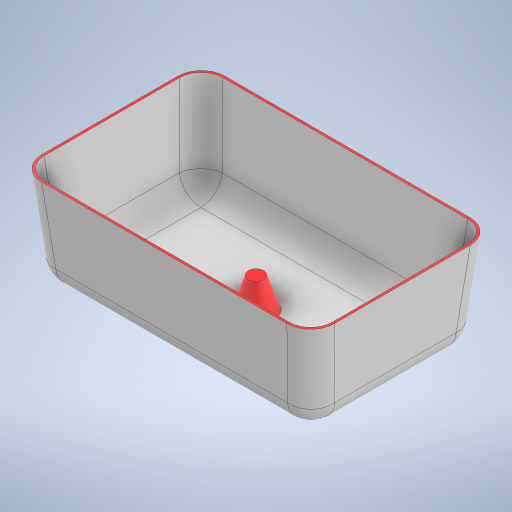
# Autodesk Inventor part: ContenedorBase
Saved by Autodesk Inventor 2024 (Build 280153000, 153)
## iProperties
Created: 2024-05-29
Part Number: ContenedorBase
Material: Genérico
Document SubType Name: Modeling
Designer: alexa
Density: 1 g/cm^3
Appearance: Valor por defecto
Author: alexa
Autodesk Inventor part; units mm, degrees
ref_plane "YZ Plane" through (0, 0, 0) normal (1, 0, 0) x (0, 1, 0)
sketch "Sketch1" plane through (0, 0, 0) normal (0, 1, 0) x (-1, 0, 0)
  line L0 (-57.75, 34.55) -> (57.75, 34.55)
  line L1 (57.75, 34.55) -> (57.75, -34.55)
  line L2 (57.75, -34.55) -> (-57.75, -34.55)
  line L3 (-57.75, -34.55) -> (-57.75, 34.55)
  line L4 (-57.75, 34.55) -> (57.75, -34.55) construction
  line L5 (57.75, 34.55) -> (-57.75, -34.55) construction
  point P0 (0, 0)
  dimension "d0" = 115.5
  dimension "d1" = 69.1
  constraints: 12 end point, 2 midpoint, 2 parallel, 1 horizontal, 1 perpendicular
  measures "d0" distance of L1.end L2.end
  measures "d1" distance of L0.end L1.end
ref_plane "Work Plane1" through (0, 40.8, 0) normal (0, 1, 0) x (-1, 0, 0)
sketch "Sketch2" plane through (0, 40.8, 0) normal (0, 1, 0) x (-1, 0, 0)
  line L0 (-61.45, 38.5) -> (61.45, 38.5)
  line L1 (61.45, 38.5) -> (61.45, -38.5)
  line L2 (61.45, -38.5) -> (-61.45, -38.5)
  line L3 (-61.45, -38.5) -> (-61.45, 38.5)
  line L4 (-61.45, 38.5) -> (61.45, -38.5) construction
  line L5 (61.45, 38.5) -> (-61.45, -38.5) construction
  point P0 (0, 0)
  dimension "d3" = 122.9
  dimension "d4" = 77
  constraints: 12 end point, 2 midpoint, 2 parallel, 1 horizontal, 1 perpendicular
  measures "d3" distance of L1.end L2.end
  measures "d4" distance of L0.end L1.end
loft "Loft1" add profiles "Sketch1", "Sketch2"
fillet "Fillet1" radius 10 8 edges at (59.6, 20.4, 36.525) (59.6, 20.4, -36.525) (-59.6, 20.4, 36.525) (-59.6, 20.4, -36.525) (0, 0, -34.55) (-57.75, 0, 0) (0, 0, 34.55) (57.75, 0, 0)
shell "Shell1" thickness 1 removed faces 1 at (17.1655, 40.8, 12.8333)
sketch "Sketch3" plane through (-48.6158, 1, -25.4714) normal (0, 1, 0) x (1, 0, 0)
  circle A0 centre (48.6158, -25.4714) radius 7.5
  dimension "d11" = 15
  constraints: 1 centre point, 1 coincident
  measures "d11" diameter of A0
ref_plane "Work Plane2" through (-48.6158, 13.5, -25.4714) normal (0, 1, 0) x (1, 0, 0)
sketch "Sketch4" plane through (-48.6158, 13.5, -25.4714) normal (0, 1, 0) x (1, 0, 0)
  circle A0 centre (48.6158, -25.4714) radius 3.25
  dimension "d13" = 6.5
  constraints: 1 centre point, 1 coincident
  measures "d13" diameter of A0
loft "Loft2" add profiles "Sketch3", "Sketch4"
body "Solid1"
